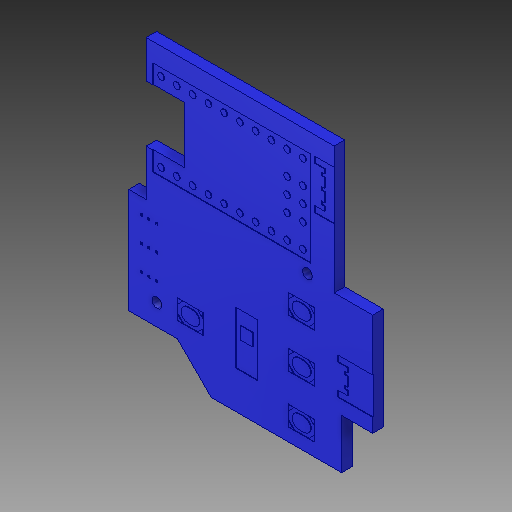
# Autodesk Inventor part: HbBoard
Saved by Autodesk Inventor 2018.1 (Build 221171000, 171)
## iProperties
Part Number: HbBoard
Material: 一般
Document SubType Name: Modeling
Designer: sktom
Density: 1 g/cm^3
Appearance: 青 - 壁塗料 - 光沢
Author: sktom
Autodesk Inventor part; units mm, degrees
ref_plane "YZ Plane" through (0, 0, 0) normal (1, 0, 0) x (0, 1, 0)
ref_plane "XZ Plane" through (0, 0, 0) normal (0, 1, 0) x (-1, 0, 0)
ref_plane "XY Plane" through (0, 0, 0) normal (0, 0, 1) x (1, 0, 0)
sketch "スケッチ1" plane through (0, 0, 0) normal (0, 0, 1) x (1, 0, 0)
  line L0 (-28.6522, -22.804) -> (-22.3388, -22.804) construction
  line L1 (-22.3388, -22.804) -> (-22.3388, -18.1815) construction
  line L2 (-22.3388, -18.1815) -> (-28.6523, -18.1815) construction
  line L3 (-28.6523, -18.1815) -> (-28.6522, -22.804) construction
  circle A0 centre (-24.112, -19.4028) radius 0.5865 construction
  line L4 (-2.2763, -1.725) -> (-2.2763, -4.725) construction
  line L5 (-2.2763, -10.7365) -> (-2.2763, -4.725) construction
  line L6 (-2.2763, -10.7365) -> (2.5447, -10.7365) construction
  line L7 (2.5448, -4.725) -> (2.5447, -10.7365) construction
  line L8 (5.4337, 19.803) -> (5.4337, -0.1035) construction
  line L9 (8.2973, 19.803) -> (5.4337, 19.803) construction
  line L10 (8.2973, 19.803) -> (8.2973, 2.3858) construction
  line L11 (8.2973, 2.3858) -> (7.6738, 2.5529) construction
  ellipse E0 centre (11.2988, 5.779) end of major axis (8.1168, -18.3905) minor radius 3.2094 (7.6738, 2.5529) -> (7.3986, -0.1035) ccw construction
  line L12 (7.3986, -0.1035) -> (5.4337, -0.1035) construction
  line L13 (4.5855, 17.733) -> (-6.16, 17.733) construction
  line L14 (-6.16, 17.733) -> (-17.5935, 17.733) construction
  line L15 (-17.5935, 17.733) -> (-29.1352, 17.733) construction
  spline S0 degree 3 poles (-29.1353, 17.1083) (-29.6143, 16.5272) (-30.1025, 15.9314) (-31.7478, 13.8487) (-32.779, 12.4115) (-34.6914, 9.373) (-35.5322, 7.8351) (-36.9922, 4.7808) (-37.6126, 3.2629) (-38.0872, 1.8206) knots 0.466857 0.466857 0.466857 0.466857 0.772898 0.772898 1.499663 1.499663 2.236131 2.236131 2.977979 2.977979 2.977979 2.977979 construction
  line L16 (-29.5527, 1.5708) -> (-29.5527, -36.2283) construction
  spline S1 degree 3 poles (-29.1127, 5.883) (-29.1127, 6.9607) (-29.1127, 8.0217) (-29.1127, 8.6087) (-29.1127, 9.1968) (-29.1127, 9.2906) (-29.1127, 8.8495) (-29.1127, 8.7808) (-29.1127, 8.7002) (-29.1127, 8.6087) (-29.1127, 8.0217) (-29.1127, 6.9607) (-29.1127, 5.883) knots -1 -1 -1 -1 -0.683333 -0.683333 -0.683333 -0.366056 -0.366056 -0.366056 -0.316667 -0.316667 -0.316667 0 0 0 0 construction
  line L17 (-15.4362, -34.0665) -> (-15.4362, -11.4365) construction
  line L18 (-15.4362, -34.0665) -> (-4.5962, -34.0665) construction
  line L19 (-4.5963, -38.9065) -> (-4.5962, -34.0665) construction
  line L20 (-4.5963, -38.9065) -> (-2.2763, -38.9065) construction
  line L21 (-2.2762, -34.0665) -> (-2.2763, -38.9065) construction
  line L22 (-2.2762, -34.0665) -> (1.7837, -34.0665) construction
  line L23 (1.7838, -11.4365) -> (1.7837, -34.0665) construction
  line L24 (1.7838, -11.4365) -> (-2.2762, -11.4365) construction
  line L25 (-2.2762, -6.5965) -> (-2.2762, -11.4365) construction
  line L26 (-4.5962, -6.5965) -> (-2.2762, -6.5965) construction
  line L27 (-4.5962, -11.4365) -> (-4.5962, -6.5965) construction
  line L28 (-4.5962, -11.4365) -> (-15.4362, -11.4365) construction
  line L29 (-15.4362, -34.0665) -> (-15.4362, -11.4365) construction
  line L30 (-15.4362, -11.4365) -> (-20.9362, -11.4365) construction
  line L31 (-20.9362, -34.0665) -> (-20.9362, -11.4365) construction
  line L32 (-20.9362, -34.0665) -> (-15.4362, -34.0665) construction
  spline S2 degree 3 poles (7.2714, -33.4077) (6.9681, -33.4081) (6.668, -33.4298) (6.3719, -33.4744) (5.9371, -33.5398) (5.5099, -33.6549) (5.0892, -33.8159) (4.6672, -33.9775) (4.2516, -34.1853) (3.8394, -34.4301) (3.381, -34.7024) (2.928, -35.0197) (2.4786, -35.36) (1.9351, -35.7716) (1.3892, -36.2222) (0.8425, -36.6629) (0.2955, -37.1038) (-0.2611, -37.5415) (-0.8412, -37.9413) (-1.2269, -38.2072) (-1.6235, -38.4567) (-2.0345, -38.68) (-2.4446, -38.9027) (-2.869, -39.0994) (-3.3087, -39.2617) (-3.7005, -39.4063) (-4.1048, -39.5234) (-4.518, -39.6095) (-4.7758, -39.6631) (-5.0379, -39.7048) (-5.3012, -39.7342) (-5.3108, -39.7352) (-5.3204, -39.7363) (-5.3299, -39.7373) knots 10.531428 10.531428 10.531428 10.531428 14.175466 14.175466 14.175466 19.526667 19.526667 19.526667 24.893879 24.893879 24.893879 30.861347 30.861347 30.861347 38.077546 38.077546 38.077546 45.296858 45.296858 45.296858 50.098281 50.098281 50.098281 54.888769 54.888769 54.888769 59.156793 59.156793 59.156793 61.818966 61.818966 61.818966 61.915662 61.915662 61.915662 61.915662 construction
  line L33 (-28.8363, -25.7715) -> (-28.8363, -23.7015) construction
  line L34 (-28.8363, -23.7015) -> (-21.3383, -23.7015) construction
  line L35 (-21.3383, -23.7015) -> (-14.7833, -30.2565) construction
  line L36 (-14.7833, -30.2565) -> (5.2957, -30.2565) construction
  line L37 (5.2957, -30.2565) -> (5.2957, -32.3265) construction
  line L38 (5.2957, -32.3265) -> (-15.6802, -32.3265) construction
  line L39 (-15.6802, -32.3265) -> (-22.2353, -25.7715) construction
  line L40 (-28.8363, -25.7715) -> (-22.2353, -25.7715) construction
  circle A1 centre (2.3288, -0.345) radius 0.8
  circle A2 centre (-24.112, -19.4028) radius 0.8
  line L41 (-28.6522, -22.804) -> (-28.6522, -5.867)
  line L42 (-28.6522, -5.867) -> (-25.8627, -5.867)
  line L43 (-25.8627, -5.867) -> (-25.8627, 16.733)
  line L44 (-25.8627, 16.733) -> (5.9172, 16.733)
  line L45 (5.9172, 16.733) -> (5.9172, -3.76)
  line L46 (6.9172, -2.76) -> (10.0274, -2.76) construction
  line L47 (11.6437, -2.76) -> (11.6437, -7.2923) construction
  line L48 (11.6437, -10.3927) -> (11.6437, -2.76) construction
  line L49 (11.2987, -28.1865) -> (11.2987, -18.5265) construction
  line L50 (5.9172, -3.76) -> (10.6437, -3.76)
  line L51 (10.6437, -3.76) -> (10.6437, -28.2565)
  line L52 (10.6437, -28.2565) -> (-15.369, -28.2565)
  line L53 (-15.369, -28.2565) -> (-20.8215, -22.804)
  line L54 (-20.8215, -22.804) -> (-28.6522, -22.804)
  line L55 (-25.8627, 2.2888) -> (-25.8627, 16.733) construction
  line L56 (-8.1718, -5.867) -> (-25.3627, -5.867) construction
  line L57 (6.9172, -2.76) -> (6.9172, 11.3672) construction
  circle A3 centre (0.1342, -3.225) radius 0.55
  line L58 (-2.2763, -4.725) -> (2.5448, -4.725)
  line L59 (2.5448, -4.725) -> (2.5447, -1.725)
  line L60 (2.5448, -4.725) -> (-2.2763, -4.725)
  line L61 (2.5447, -1.725) -> (-2.2763, -1.725)
  point P0 (0, 0)
  point P1 (-17.9831, -31.2915)
  dimension "d0" = 1.6
  dimension "d1" = 1.6
  dimension "d3" = 1
  dimension "d4" = 1
  dimension "d5" = 1
  dimension "d6" = 1
  dimension "d7" = 2
  dimension "d8" = 1
  constraints: 20 end point, 3 horizontal, 3 parallel, 2 centre point, 2 perpendicular, 1 coincident, 1 horizontal alignment, 1 vertical, 1 vertical alignment, 2 other
  measures "d0" diameter of A1
  measures "d1" diameter of A2
  measures "d3" distance between parallel lines of L44 L15
  measures "d4" distance between parallel lines of L57 L45
  measures "d5" distance between parallel lines of L46 L50
  measures "d6" distance between parallel lines of L48 L51
  measures "d7" distance between parallel lines of L36 L52
  measures "d8" distance between parallel lines of L35 L53
extrude "押し出し1" add sketch "スケッチ1" along normal blind 1.7 contours L41 L42 L43 L44 L45 L50 L51 L52 L53 L54 | A3
sketch "スケッチ2" plane through (0, 0, 1.7) normal (0, 0, 1) x (1, 0, 0)
  line L0 (10.6437, -28.2565) -> (10.6437, -3.76) projected
  line L1 (10.6437, -28.2565) -> (5.6437, -28.2565)
  line L2 (10.6437, -28.2565) -> (-15.369, -28.2565) projected
  line L3 (5.6437, -28.2565) -> (5.6437, -20.2565)
  line L4 (5.6437, -20.2565) -> (10.6437, -20.2565)
  line L5 (10.6437, -20.2565) -> (10.6437, -28.2565)
  point P0 (0, 0)
  dimension "d11" = 8
  dimension "d12" = 5
  constraints: 8 end point, 1 horizontal, 1 parallel, 1 point on line, 1 vertical
  measures "d11" distance of L1.end L3.end
  measures "d12" distance of L0.start L1.end
extrude "押し出し2" cut sketch "スケッチ2" against normal blind 1.7
sketch "スケッチ3" plane through (0, 0, 1.7) normal (0, 0, 1) x (1, 0, 0)
  circle A0 centre (0.1342, -3.225) radius 0.55 construction
  circle A1 centre (0.1342, -3.225) radius 0.8
  point P0 (0, 0)
  dimension "d15" = 1.6
  constraints: 1 centre point, 1 coincident
  measures "d15" diameter of A1
extrude "押し出し3" cut sketch "スケッチ3" against normal blind 1.7
delete faces "削除1" heal yes whole lump no faces at (3.1262, -0.4094, 1.1333)
sketch "スケッチ4" plane through (-25.8627, 16.733, 1.7) normal (0, 0, 1) x (1, 0, 0)
  circle A0 centre (5.81, -8.08) radius 0.51 construction
  circle A1 centre (5.81, -10.62) radius 0.51 construction
  circle A2 centre (5.81, -13.16) radius 0.51 construction
  circle A3 centre (5.81, -4.27) radius 0.51 construction
  circle A4 centre (10.89, -4.27) radius 0.51 construction
  circle A5 centre (15.97, -4.27) radius 0.51 construction
  circle A6 centre (21.05, -4.27) radius 0.51 construction
  circle A7 centre (26.13, -4.27) radius 0.51 construction
  circle A8 centre (5.81, -16.97) radius 0.51 construction
  circle A9 centre (10.89, -16.97) radius 0.51 construction
  circle A10 centre (15.97, -16.97) radius 0.51 construction
  circle A11 centre (21.05, -16.97) radius 0.51 construction
  circle A12 centre (26.13, -16.97) radius 0.51 construction
  circle A13 centre (23.59, -16.97) radius 0.51 construction
  circle A14 centre (18.51, -16.97) radius 0.51 construction
  circle A15 centre (13.43, -16.97) radius 0.51 construction
  circle A16 centre (8.35, -16.97) radius 0.51 construction
  circle A17 centre (3.27, -16.97) radius 0.51 construction
  circle A18 centre (23.59, -4.27) radius 0.51 construction
  circle A19 centre (18.51, -4.27) radius 0.51 construction
  circle A20 centre (13.43, -4.27) radius 0.51 construction
  circle A21 centre (8.35, -4.27) radius 0.51 construction
  circle A22 centre (3.27, -4.27) radius 0.51 construction
  circle A23 centre (3.27, -13.16) radius 0.51 construction
  circle A24 centre (3.27, -10.62) radius 0.51 construction
  circle A25 centre (3.27, -8.08) radius 0.51 construction
  line L0 (2, -18.24) -> (2, -3) construction
  line L1 (27.4, -18.24) -> (2, -18.24) construction
  line L2 (27.4, -3) -> (27.4, -18.24) construction
  line L3 (2, -3) -> (27.4, -3) construction
  line L4 (27.4, -6.57) -> (27.4, -14.67) construction
  line L5 (28.5, -14.67) -> (27.4, -14.67) construction
  line L6 (28.5, -6.57) -> (28.5, -14.67) construction
  line L7 (27.4, -6.57) -> (28.5, -6.57) construction
  line L8 (22.9, -14.67) -> (27.4, -14.67) construction
  line L9 (22.9, -6.57) -> (22.9, -14.67) construction
  line L10 (31.78, -17.07) -> (28, -17.07)
  line L11 (28, -17.07) -> (28, -15.07)
  line L12 (28, -15.07) -> (22.5, -15.07)
  line L13 (22.5, -15.07) -> (22.5, -6.17)
  line L14 (22.5, -6.17) -> (28, -6.17)
  line L15 (28, -6.17) -> (28, 0)
  line L16 (31.78, 0) -> (0, 0) projected
  line L17 (31.78, 0) -> (31.78, -17.07)
  point P0 (25.8627, -16.733)
  dimension "d18" = 0.4
  dimension "d19" = 0.4
  dimension "d20" = 0.4
  dimension "d21" = 0.6
  dimension "d22" = 2
  constraints: 14 end point, 5 perpendicular, 3 point on line, 1 horizontal
  measures "d18" distance between parallel lines of L8 L12
  measures "d19" distance between parallel lines of L9 L13
  measures "d20" distance between parallel lines of L7 L14
  measures "d21" distance between parallel lines of L2 L15
  measures "d22" distance of L10.end L11.end
extrude "押し出し4" cut sketch "スケッチ4" against normal blind 1.7
sketch "スケッチ5" plane through (-15.369, -28.2565, 1.7) normal (0, 0, 1) x (1, 0, 0)
  line L0 (26.0128, 24.4965) -> (21.2863, 24.4965) projected
  line L1 (17.5063, 27.9195) -> (17.5063, 29.9195) projected
  line L2 (21.2863, 24.4965) -> (17.5063, 24.4965)
  line L3 (17.5063, 24.4965) -> (17.5063, 27.9195)
  line L4 (17.5063, 27.9195) -> (21.2863, 27.9195)
  line L5 (21.2863, 27.9195) -> (21.2863, 24.4965)
  point P0 (15.369, 28.2565)
  constraints: 8 end point, 2 parallel, 1 horizontal, 1 perpendicular
extrude "押し出し5" cut sketch "スケッチ5" against normal blind 1.7
sketch "スケッチ6" plane through (-15.369, -28.2565, 1.7) normal (0, 0, 1) x (1, 0, 0)
  line L0 (-10.4937, 44.9895) -> (17.5063, 44.9895) projected
  line L1 (17.5063, 44.9895) -> (19.8063, 44.9895)
  line L2 (19.8063, 44.9895) -> (19.8063, 24.4965)
  line L3 (17.5063, 24.4965) -> (26.0128, 24.4965) projected
  line L4 (17.5063, 38.8195) -> (17.5063, 44.9895) projected
  line L5 (17.5063, 29.9195) -> (17.5063, 24.4965) projected
  line L6 (19.8063, 24.4965) -> (17.5063, 24.4965)
  line L7 (17.5063, 24.4965) -> (17.5063, 29.9195)
  line L8 (12.0063, 29.9195) -> (12.0063, 38.8195) projected
  line L9 (17.5063, 29.9195) -> (12.0063, 29.9195)
  line L10 (12.0063, 29.9195) -> (12.0063, 38.8195)
  line L11 (17.5063, 38.8195) -> (12.0063, 38.8195) projected
  line L12 (12.0063, 38.8195) -> (17.5063, 38.8195)
  line L13 (17.5063, 38.8195) -> (17.5063, 44.9895)
  point P0 (15.369, 28.2565)
  dimension "d27" = 2.3
  constraints: 16 end point, 6 perpendicular, 1 collinear, 1 horizontal, 1 point on line
  measures "d27" distance between parallel lines of L4 L2
extrude "押し出し6" add sketch "スケッチ6" against normal up to surface (1.7 mm away)
sketch "スケッチ7" plane through (-15.369, -28.2565, 1.7) normal (0, 0, 1) x (1, 0, 0)
  line L0 (-9.3937, 30.3195) -> (-9.3937, 38.4195) projected
  line L1 (-10.4937, 38.4195) -> (-9.3937, 38.4195) projected
  line L2 (-10.4937, 30.3195) -> (-10.4937, 38.4195) projected
  line L3 (-9.3937, 30.3195) -> (-10.4937, 30.3195) projected
  line L4 (-4.8937, 30.3195) -> (-4.8937, 38.4195) projected
  line L5 (-10.9937, 38.9195) -> (-4.3937, 38.9195)
  line L6 (-4.3937, 38.9195) -> (-4.3937, 29.8195)
  line L7 (-4.3937, 29.8195) -> (-10.9937, 29.8195)
  line L8 (-10.9937, 29.8195) -> (-10.9937, 38.9195)
  point P0 (15.369, 28.2565)
  dimension "d30" = 0.5
  dimension "d31" = 0.5
  dimension "d32" = 0.5
  dimension "d33" = 0.5
  constraints: 8 end point, 2 parallel, 1 horizontal, 1 perpendicular
  measures "d30" distance between parallel lines of L6 L4
  measures "d31" distance between parallel lines of L3 L7
  measures "d32" distance between parallel lines of L1 L5
  measures "d33" distance between parallel lines of L2 L8
extrude "押し出し7" cut sketch "スケッチ7" against normal blind 10 contours L3 L2 L1 L0 | L5 L6 L7 L8
sketch "スケッチ8" plane through (-15.369, -28.2565, 1.7) normal (0, 0, 1) x (1, 0, 0)
  line L0 (22.0128, 11.93) -> (21.5128, 11.93) projected
  line L1 (22.0128, 12.43) -> (22.0128, 11.93) projected
  line L2 (21.5128, 12.43) -> (22.0128, 12.43) projected
  line L3 (21.5128, 11.93) -> (21.5128, 12.43) projected
  line L4 (22.0128, 13.93) -> (21.5128, 13.93) projected
  line L5 (22.0128, 14.43) -> (22.0128, 13.93) projected
  line L6 (21.5128, 14.43) -> (22.0128, 14.43) projected
  line L7 (21.5128, 13.93) -> (21.5128, 14.43) projected
  line L8 (16.5666, 9.924) -> (15.7166, 9.924) projected
  line L9 (15.7166, 9.924) -> (16.5666, 10.774) projected
  line L10 (16.5666, 10.774) -> (16.5666, 9.924) projected
  line L11 (13.3166, 9.924) -> (12.4666, 9.924) projected
  line L12 (12.4666, 9.924) -> (12.4666, 10.774) projected
  line L13 (12.4666, 10.774) -> (13.3166, 9.924) projected
  line L14 (15.7166, 13.024) -> (16.5666, 13.024) projected
  line L15 (16.5666, 13.024) -> (16.5666, 12.174) projected
  line L16 (16.5666, 12.174) -> (15.7166, 13.024) projected
  line L17 (12.4666, 13.024) -> (13.3166, 13.024) projected
  line L18 (13.3166, 13.024) -> (12.4666, 12.174) projected
  line L19 (12.4666, 12.174) -> (12.4666, 13.024) projected
  arc A0 (14.1166, 12.574) -> (14.1166, 10.374) centre (14.1166, 11.474) ccw projected
  line L20 (14.1166, 12.574) -> (14.9166, 12.574) projected
  arc A1 (14.9166, 10.374) -> (14.9166, 12.574) centre (14.9166, 11.474) ccw projected
  line L21 (14.9166, 10.374) -> (14.1166, 10.374) projected
  line L22 (12.4166, 9.874) -> (16.6166, 9.874) projected
  line L23 (16.6166, 9.874) -> (16.6166, 13.074) projected
  line L24 (16.6166, 13.074) -> (12.4166, 13.074) projected
  line L25 (12.4166, 13.074) -> (12.4166, 9.874) projected
  line L26 (16.5666, 2.124) -> (15.7166, 2.124) projected
  line L27 (15.7166, 2.124) -> (16.5666, 2.974) projected
  line L28 (16.5666, 2.974) -> (16.5666, 2.124) projected
  line L29 (13.3166, 2.124) -> (12.4666, 2.124) projected
  line L30 (12.4666, 2.124) -> (12.4666, 2.974) projected
  line L31 (12.4666, 2.974) -> (13.3166, 2.124) projected
  line L32 (15.7166, 5.224) -> (16.5666, 5.224) projected
  line L33 (16.5666, 5.224) -> (16.5666, 4.374) projected
  line L34 (16.5666, 4.374) -> (15.7166, 5.224) projected
  line L35 (12.4666, 5.224) -> (13.3166, 5.224) projected
  line L36 (13.3166, 5.224) -> (12.4666, 4.374) projected
  line L37 (12.4666, 4.374) -> (12.4666, 5.224) projected
  arc A2 (14.1166, 4.774) -> (14.1166, 2.574) centre (14.1166, 3.674) ccw projected
  line L38 (14.1166, 4.774) -> (14.9166, 4.774) projected
  arc A3 (14.9166, 2.574) -> (14.9166, 4.774) centre (14.9166, 3.674) ccw projected
  line L39 (14.9166, 2.574) -> (14.1166, 2.574) projected
  line L40 (12.4166, 2.074) -> (16.6166, 2.074) projected
  line L41 (16.6166, 2.074) -> (16.6166, 5.274) projected
  line L42 (16.6166, 5.274) -> (12.4166, 5.274) projected
  line L43 (12.4166, 5.274) -> (12.4166, 2.074) projected
  line L44 (16.5666, 17.724) -> (15.7166, 17.724) projected
  line L45 (15.7166, 17.724) -> (16.5666, 18.574) projected
  line L46 (16.5666, 18.574) -> (16.5666, 17.724) projected
  line L47 (13.3166, 17.724) -> (12.4666, 17.724) projected
  line L48 (12.4666, 17.724) -> (12.4666, 18.574) projected
  line L49 (12.4666, 18.574) -> (13.3166, 17.724) projected
  line L50 (15.7166, 20.824) -> (16.5666, 20.824) projected
  line L51 (16.5666, 20.824) -> (16.5666, 19.974) projected
  line L52 (16.5666, 19.974) -> (15.7166, 20.824) projected
  line L53 (12.4666, 20.824) -> (13.3166, 20.824) projected
  line L54 (13.3166, 20.824) -> (12.4666, 19.974) projected
  line L55 (12.4666, 19.974) -> (12.4666, 20.824) projected
  arc A4 (14.1166, 20.374) -> (14.1166, 18.174) centre (14.1166, 19.274) ccw projected
  line L56 (14.1166, 20.374) -> (14.9166, 20.374) projected
  arc A5 (14.9166, 18.174) -> (14.9166, 20.374) centre (14.9166, 19.274) ccw projected
  line L57 (14.9166, 18.174) -> (14.1166, 18.174) projected
  line L58 (12.4166, 17.674) -> (16.6166, 17.674) projected
  line L59 (16.6166, 17.674) -> (16.6166, 20.874) projected
  line L60 (16.6166, 20.874) -> (12.4166, 20.874) projected
  line L61 (12.4166, 20.874) -> (12.4166, 17.674) projected
  line L62 (-1.2944, 11.1885) -> (-5.4944, 11.1885) projected
  line L63 (-1.3444, 8.0385) -> (-2.1944, 8.0385) projected
  line L64 (-2.1944, 8.0385) -> (-1.3444, 8.8885) projected
  line L65 (-1.3444, 8.8885) -> (-1.3444, 8.0385) projected
  line L66 (-4.5944, 8.0385) -> (-5.4444, 8.0385) projected
  line L67 (-5.4444, 8.0385) -> (-5.4444, 8.8885) projected
  line L68 (-5.4444, 8.8885) -> (-4.5944, 8.0385) projected
  line L69 (-2.1944, 11.1385) -> (-1.3444, 11.1385) projected
  line L70 (-1.3444, 11.1385) -> (-1.3444, 10.2885) projected
  line L71 (-1.3444, 10.2885) -> (-2.1944, 11.1385) projected
  line L72 (-5.4444, 11.1385) -> (-4.5944, 11.1385) projected
  line L73 (-4.5944, 11.1385) -> (-5.4444, 10.2885) projected
  line L74 (-5.4444, 10.2885) -> (-5.4444, 11.1385) projected
  arc A6 (-3.7944, 10.6885) -> (-3.7944, 8.4885) centre (-3.7944, 9.5885) ccw projected
  line L75 (-3.7944, 10.6885) -> (-2.9944, 10.6885) projected
  arc A7 (-2.9944, 8.4885) -> (-2.9944, 10.6885) centre (-2.9944, 9.5885) ccw projected
  line L76 (-2.9944, 8.4885) -> (-3.7944, 8.4885) projected
  line L77 (-5.4944, 7.9885) -> (-1.2944, 7.9885) projected
  line L78 (-1.2944, 7.9885) -> (-1.2944, 11.1885) projected
  line L79 (-1.2944, 11.1885) -> (-5.4944, 11.1885) projected
  line L80 (-5.4944, 11.1885) -> (-5.4944, 7.9885) projected
  line L81 (4.6778, 10.3689) -> (4.6778, 12.3689) projected
  line L82 (4.6778, 12.3689) -> (6.6778, 12.3689) projected
  line L83 (6.6778, 12.3689) -> (6.6778, 10.3689) projected
  line L84 (6.6778, 10.3689) -> (4.6778, 10.3689) projected
  line L85 (3.9278, 6.0689) -> (7.4278, 6.0689) projected
  line L86 (7.4278, 6.0689) -> (7.4278, 14.5689) projected
  line L87 (7.4278, 14.5689) -> (3.9278, 14.5689) projected
  line L88 (3.9278, 14.5689) -> (3.9278, 6.0689) projected
  circle A8 centre (12.1963, 31.8295) radius 0.51 projected
  circle A9 centre (12.1963, 34.3695) radius 0.51 projected
  circle A10 centre (12.1963, 36.9095) radius 0.51 projected
  circle A11 centre (12.1963, 28.0195) radius 0.51 projected
  circle A12 centre (7.1163, 28.0195) radius 0.51 projected
  circle A13 centre (2.0363, 28.0195) radius 0.51 projected
  circle A14 centre (-3.0437, 28.0195) radius 0.51 projected
  circle A15 centre (-8.1237, 28.0195) radius 0.51 projected
  circle A16 centre (12.1963, 40.7195) radius 0.51 projected
  circle A17 centre (7.1163, 40.7195) radius 0.51 projected
  circle A18 centre (2.0363, 40.7195) radius 0.51 projected
  circle A19 centre (-3.0437, 40.7195) radius 0.51 projected
  circle A20 centre (-8.1237, 40.7195) radius 0.51 projected
  circle A21 centre (-5.5837, 40.7195) radius 0.51 projected
  circle A22 centre (-0.5037, 40.7195) radius 0.51 projected
  circle A23 centre (4.5763, 40.7195) radius 0.51 projected
  circle A24 centre (9.6563, 40.7195) radius 0.51 projected
  circle A25 centre (14.7363, 40.7195) radius 0.51 projected
  circle A26 centre (-5.5837, 28.0195) radius 0.51 projected
  circle A27 centre (-0.5037, 28.0195) radius 0.51 projected
  circle A28 centre (4.5763, 28.0195) radius 0.51 projected
  circle A29 centre (9.6563, 28.0195) radius 0.51 projected
  circle A30 centre (14.7363, 28.0195) radius 0.51 projected
  circle A31 centre (14.7363, 36.9095) radius 0.51 projected
  circle A32 centre (14.7363, 34.3695) radius 0.51 projected
  circle A33 centre (14.7363, 31.8295) radius 0.51 projected
  line L89 (16.0063, 41.9895) -> (16.0063, 26.7495) projected
  line L90 (-9.3937, 41.9895) -> (16.0063, 41.9895) projected
  line L91 (-9.3937, 26.7495) -> (-9.3937, 41.9895) projected
  line L92 (16.0063, 26.7495) -> (-9.3937, 26.7495) projected
  line L93 (18.2863, 35.821) -> (17.7863, 35.821) projected
  line L94 (18.2863, 36.321) -> (18.2863, 35.821) projected
  line L95 (17.7863, 36.321) -> (18.2863, 36.321) projected
  line L96 (17.7863, 35.821) -> (17.7863, 36.321) projected
  line L97 (18.2863, 37.821) -> (17.7863, 37.821) projected
  line L98 (18.2863, 38.321) -> (18.2863, 37.821) projected
  line L99 (17.7863, 38.321) -> (18.2863, 38.321) projected
  line L100 (17.7863, 37.821) -> (17.7863, 38.321) projected
  line L101 (18.7328, 29.2915) -> (18.7328, 45.9895) projected
  line L102 (18.2863, 39.821) -> (17.7863, 39.821) projected
  line L103 (18.2863, 40.321) -> (18.2863, 39.821) projected
  line L104 (17.7863, 40.321) -> (18.2863, 40.321) projected
  line L105 (17.7863, 39.821) -> (17.7863, 40.321) projected
  line L106 (18.2863, 41.021) -> (18.2863, 40.321) projected
  line L107 (18.2863, 40.321) -> (18.2863, 39.821) projected
  line L108 (18.2863, 39.821) -> (18.2863, 38.321) projected
  line L109 (18.2863, 38.321) -> (18.2863, 37.821) projected
  line L110 (18.2863, 37.821) -> (18.2863, 36.321) projected
  line L111 (18.2863, 36.321) -> (18.2863, 35.821) projected
  line L112 (18.2863, 35.821) -> (18.2863, 35.121) projected
  line L113 (18.2863, 35.121) -> (16.6863, 35.121) projected
  line L114 (16.6863, 34.121) -> (16.6863, 35.121) projected
  line L115 (24.2863, 34.121) -> (16.6863, 34.121) projected
  line L116 (24.2863, 34.121) -> (24.2863, 42.021) projected
  line L117 (24.2863, 42.021) -> (16.6863, 42.021) projected
  line L118 (16.6863, 41.021) -> (16.6863, 42.021) projected
  line L119 (16.6863, 41.021) -> (18.2863, 41.021) projected
  line L120 (-11.4432, 20.0251) -> (-11.3332, 19.9151) projected
  line L121 (-11.4432, 20.0251) -> (-11.4432, 19.6751) projected
  line L122 (-11.4432, 19.6751) -> (-11.3332, 19.7851) projected
  line L123 (-11.3332, 19.9151) -> (-11.3332, 19.7851) projected
  line L124 (-11.4432, 20.0251) -> (-11.3332, 19.9151) projected
  line L125 (-11.2332, 19.9151) -> (-11.3332, 19.9151) projected
  line L126 (-11.1232, 20.0251) -> (-11.2332, 19.9151) projected
  line L127 (-11.1232, 20.0251) -> (-11.4432, 20.0251) projected
  line L128 (-11.1232, 20.0251) -> (-11.2332, 19.9151) projected
  line L129 (-11.2332, 19.7851) -> (-11.2332, 19.9151) projected
  line L130 (-11.1232, 19.6751) -> (-11.2332, 19.7851) projected
  line L131 (-11.1232, 19.6751) -> (-11.1232, 20.0251) projected
  line L132 (-11.4432, 19.6751) -> (-11.3332, 19.7851) projected
  line L133 (-11.4432, 19.6751) -> (-11.1232, 19.6751) projected
  line L134 (-11.1232, 19.6751) -> (-11.2332, 19.7851) projected
  line L135 (-11.3332, 19.7851) -> (-11.2332, 19.7851) projected
  line L136 (-10.1932, 19.6751) -> (-10.0832, 19.7851) projected
  line L137 (-10.1932, 19.6751) -> (-9.8732, 19.6751) projected
  line L138 (-9.8732, 19.6751) -> (-9.9832, 19.7851) projected
  line L139 (-10.0832, 19.7851) -> (-9.9832, 19.7851) projected
  line L140 (-9.8732, 20.0251) -> (-9.9832, 19.9151) projected
  line L141 (-9.9832, 19.7851) -> (-9.9832, 19.9151) projected
  line L142 (-9.8732, 19.6751) -> (-9.9832, 19.7851) projected
  line L143 (-9.8732, 19.6751) -> (-9.8732, 20.0251) projected
  line L144 (-10.1932, 20.0251) -> (-10.0832, 19.9151) projected
  line L145 (-10.1932, 20.0251) -> (-10.1932, 19.6751) projected
  line L146 (-10.1932, 19.6751) -> (-10.0832, 19.7851) projected
  line L147 (-10.0832, 19.9151) -> (-10.0832, 19.7851) projected
  line L148 (-10.1932, 20.0251) -> (-10.0832, 19.9151) projected
  line L149 (-9.9832, 19.9151) -> (-10.0832, 19.9151) projected
  line L150 (-9.8732, 20.0251) -> (-9.9832, 19.9151) projected
  line L151 (-9.8732, 20.0251) -> (-10.1932, 20.0251) projected
  line L152 (-8.9432, 19.6751) -> (-8.6232, 19.6751) projected
  line L153 (-8.6232, 19.6751) -> (-8.7332, 19.7851) projected
  line L154 (-8.8332, 19.7851) -> (-8.7332, 19.7851) projected
  line L155 (-8.9432, 19.6751) -> (-8.8332, 19.7851) projected
  line L156 (-8.9432, 20.0251) -> (-8.9432, 19.6751) projected
  line L157 (-8.9432, 19.6751) -> (-8.8332, 19.7851) projected
  line L158 (-8.8332, 19.9151) -> (-8.8332, 19.7851) projected
  line L159 (-8.9432, 20.0251) -> (-8.8332, 19.9151) projected
  line L160 (-8.7332, 19.7851) -> (-8.7332, 19.9151) projected
  line L161 (-8.6232, 19.6751) -> (-8.7332, 19.7851) projected
  line L162 (-8.6232, 19.6751) -> (-8.6232, 20.0251) projected
  line L163 (-8.6232, 20.0251) -> (-8.7332, 19.9151) projected
  line L164 (-8.7332, 19.9151) -> (-8.8332, 19.9151) projected
  line L165 (-8.6232, 20.0251) -> (-8.7332, 19.9151) projected
  line L166 (-8.6232, 20.0251) -> (-8.9432, 20.0251) projected
  line L167 (-8.9432, 20.0251) -> (-8.8332, 19.9151) projected
  line L168 (-8.9432, 15.6751) -> (-8.6232, 15.6751) projected
  line L169 (-8.6232, 15.6751) -> (-8.7332, 15.7851) projected
  line L170 (-8.8332, 15.7851) -> (-8.7332, 15.7851) projected
  line L171 (-8.9432, 15.6751) -> (-8.8332, 15.7851) projected
  line L172 (-8.7332, 15.7851) -> (-8.7332, 15.9151) projected
  line L173 (-8.6232, 15.6751) -> (-8.7332, 15.7851) projected
  line L174 (-8.6232, 15.6751) -> (-8.6232, 16.0251) projected
  line L175 (-8.6232, 16.0251) -> (-8.7332, 15.9151) projected
  line L176 (-8.7332, 15.9151) -> (-8.8332, 15.9151) projected
  line L177 (-8.6232, 16.0251) -> (-8.7332, 15.9151) projected
  line L178 (-8.6232, 16.0251) -> (-8.9432, 16.0251) projected
  line L179 (-8.9432, 16.0251) -> (-8.8332, 15.9151) projected
  line L180 (-8.9432, 16.0251) -> (-8.9432, 15.6751) projected
  line L181 (-8.9432, 15.6751) -> (-8.8332, 15.7851) projected
  line L182 (-8.8332, 15.9151) -> (-8.8332, 15.7851) projected
  line L183 (-8.9432, 16.0251) -> (-8.8332, 15.9151) projected
  line L184 (-9.8732, 16.0251) -> (-9.9832, 15.9151) projected
  line L185 (-9.9832, 15.7851) -> (-9.9832, 15.9151) projected
  line L186 (-9.8732, 15.6751) -> (-9.9832, 15.7851) projected
  line L187 (-9.8732, 15.6751) -> (-9.8732, 16.0251) projected
  line L188 (-10.1932, 15.6751) -> (-10.0832, 15.7851) projected
  line L189 (-10.1932, 15.6751) -> (-9.8732, 15.6751) projected
  line L190 (-9.8732, 15.6751) -> (-9.9832, 15.7851) projected
  line L191 (-10.0832, 15.7851) -> (-9.9832, 15.7851) projected
  line L192 (-9.9832, 16.0251) -> (-9.9832, 15.6251) projected
  line L193 (-10.1932, 16.0251) -> (-10.0832, 15.9151) projected
  line L194 (-9.9832, 15.9151) -> (-10.0832, 15.9151) projected
  line L195 (-9.8732, 16.0251) -> (-9.9832, 15.9151) projected
  line L196 (-9.8732, 16.0251) -> (-10.1932, 16.0251) projected
  line L197 (-10.1932, 16.0251) -> (-10.0832, 15.9151) projected
  line L198 (-10.1932, 16.0251) -> (-10.1932, 15.6751) projected
  line L199 (-10.1932, 15.6751) -> (-10.0832, 15.7851) projected
  line L200 (-10.0832, 15.9151) -> (-10.0832, 15.7851) projected
  line L201 (-11.1232, 16.0251) -> (-11.2332, 15.9151) projected
  line L202 (-11.2332, 15.7851) -> (-11.2332, 15.9151) projected
  line L203 (-11.1232, 15.6751) -> (-11.2332, 15.7851) projected
  line L204 (-11.1232, 15.6751) -> (-11.1232, 16.0251) projected
  line L205 (-11.4432, 15.6751) -> (-11.3332, 15.7851) projected
  line L206 (-11.4432, 15.6751) -> (-11.1232, 15.6751) projected
  line L207 (-11.1232, 15.6751) -> (-11.2332, 15.7851) projected
  line L208 (-11.3332, 15.7851) -> (-11.2332, 15.7851) projected
  line L209 (-11.4432, 16.0251) -> (-11.3332, 15.9151) projected
  line L210 (-11.4432, 16.0251) -> (-11.4432, 15.6751) projected
  line L211 (-11.4432, 15.6751) -> (-11.3332, 15.7851) projected
  line L212 (-11.3332, 15.9151) -> (-11.3332, 15.7851) projected
  line L213 (-11.4432, 16.0251) -> (-11.3332, 15.9151) projected
  line L214 (-11.2332, 15.9151) -> (-11.3332, 15.9151) projected
  line L215 (-11.1232, 16.0251) -> (-11.2332, 15.9151) projected
  line L216 (-11.1232, 16.0251) -> (-11.4432, 16.0251) projected
  line L217 (-11.4432, 11.6751) -> (-11.3332, 11.7851) projected
  line L218 (-11.4432, 11.6751) -> (-11.1232, 11.6751) projected
  line L219 (-11.1232, 11.6751) -> (-11.2332, 11.7851) projected
  line L220 (-11.3332, 11.7851) -> (-11.2332, 11.7851) projected
  line L221 (-11.4432, 12.0251) -> (-11.3332, 11.9151) projected
  line L222 (-11.4432, 12.0251) -> (-11.4432, 11.6751) projected
  line L223 (-11.4432, 11.6751) -> (-11.3332, 11.7851) projected
  line L224 (-11.3332, 11.9151) -> (-11.3332, 11.7851) projected
  line L225 (-11.4432, 12.0251) -> (-11.3332, 11.9151) projected
  line L226 (-11.2332, 11.9151) -> (-11.3332, 11.9151) projected
  line L227 (-11.1232, 12.0251) -> (-11.2332, 11.9151) projected
  line L228 (-11.1232, 12.0251) -> (-11.4432, 12.0251) projected
  line L229 (-11.1232, 12.0251) -> (-11.2332, 11.9151) projected
  line L230 (-11.2332, 11.7851) -> (-11.2332, 11.9151) projected
  line L231 (-11.1232, 11.6751) -> (-11.2332, 11.7851) projected
  line L232 (-11.1232, 11.6751) -> (-11.1232, 12.0251) projected
  line L233 (-10.1932, 12.0251) -> (-10.0832, 11.9151) projected
  line L234 (-10.1932, 12.0251) -> (-10.1932, 11.6751) projected
  line L235 (-10.1932, 11.6751) -> (-10.0832, 11.7851) projected
  line L236 (-10.0832, 11.9151) -> (-10.0832, 11.7851) projected
  line L237 (-10.1932, 11.6751) -> (-10.0832, 11.7851) projected
  line L238 (-10.1932, 11.6751) -> (-9.8732, 11.6751) projected
  line L239 (-9.8732, 11.6751) -> (-9.9832, 11.7851) projected
  line L240 (-10.0832, 11.7851) -> (-9.9832, 11.7851) projected
  line L241 (-10.1932, 12.0251) -> (-10.0832, 11.9151) projected
  line L242 (-9.9832, 11.9151) -> (-10.0832, 11.9151) projected
  line L243 (-9.8732, 12.0251) -> (-9.9832, 11.9151) projected
  line L244 (-9.8732, 12.0251) -> (-10.1932, 12.0251) projected
  line L245 (-9.8732, 12.0251) -> (-9.9832, 11.9151) projected
  line L246 (-9.9832, 11.7851) -> (-9.9832, 11.9151) projected
  line L247 (-9.8732, 11.6751) -> (-9.9832, 11.7851) projected
  line L248 (-9.8732, 11.6751) -> (-9.8732, 12.0251) projected
  line L249 (-8.9432, 12.0251) -> (-8.9432, 11.6751) projected
  line L250 (-8.9432, 11.6751) -> (-8.8332, 11.7851) projected
  line L251 (-8.8332, 11.9151) -> (-8.8332, 11.7851) projected
  line L252 (-8.9432, 12.0251) -> (-8.8332, 11.9151) projected
  line L253 (-8.9432, 11.6751) -> (-8.6232, 11.6751) projected
  line L254 (-8.6232, 11.6751) -> (-8.7332, 11.7851) projected
  line L255 (-8.8332, 11.7851) -> (-8.7332, 11.7851) projected
  line L256 (-8.9432, 11.6751) -> (-8.8332, 11.7851) projected
  line L257 (-8.7332, 11.7851) -> (-8.7332, 11.9151) projected
  line L258 (-8.6232, 11.6751) -> (-8.7332, 11.7851) projected
  line L259 (-8.6232, 11.6751) -> (-8.6232, 12.0251) projected
  line L260 (-8.6232, 12.0251) -> (-8.7332, 11.9151) projected
  line L261 (-8.6232, 12.0251) -> (-8.9432, 12.0251) projected
  line L262 (-8.7332, 11.9151) -> (-8.8332, 11.9151) projected
  line L263 (-8.6232, 12.0251) -> (-8.7332, 11.9151) projected
  line L264 (-8.6232, 12.0251) -> (-8.9432, 12.0251) projected
  line L265 (-8.9432, 12.0251) -> (-8.8332, 11.9151) projected
  line L266 (22.0128, 15.13) -> (22.0128, 14.43) projected
  line L267 (22.0128, 14.43) -> (22.0128, 13.93) projected
  line L268 (22.0128, 13.93) -> (22.0128, 12.43) projected
  line L269 (22.0128, 12.43) -> (22.0128, 11.93) projected
  line L270 (22.0128, 11.93) -> (22.0128, 11.23) projected
  line L271 (22.0128, 11.23) -> (20.4128, 11.23) projected
  line L272 (20.4128, 10.23) -> (20.4128, 11.23) projected
  line L273 (28.0128, 10.23) -> (20.4128, 10.23) projected
  line L274 (28.0128, 10.23) -> (28.0128, 16.13) projected
  line L275 (28.0128, 16.13) -> (20.4128, 16.13) projected
  line L276 (20.4128, 15.13) -> (20.4128, 16.13) projected
  line L277 (20.4128, 15.13) -> (22.0128, 15.13) projected
  line L278 (-12.7832, 10.7001) -> (-12.7832, 13.5001) projected
  point P0 (15.369, 28.2565)
extrude "押し出し8" cut sketch "スケッチ8" against normal blind 0.1 contours L0 L3 L2 L1 | L1 L268 L5 L266 L277 L276 L275 L274 L273 L272 L271 L270 | L4 L7 L6 L5 | L25 L24 L23 L22 | L43 L42 L41 L40 | L61 L60 L59 L58 | L78 L77 L80 L62 | L88 L87 L86 L85 | L89 L92 L91 L90 | L93 L96 L95 L94 | L94 L110 L98 L108 L103 L106 L119 L118 L117 L101 L115 L114 L113 L112 | L97 L100 L99 L98 | L102 L105 L104 L103 | L101 L117 L116 L115 | L127 L126 L125 L120 | L120 L123 L122 L121 | L122 L135 L130 L133 | L131 L130 L129 L126 | L145 L144 L147 L136 | L136 L139 L138 L137 | L138 L141 L140 L143 | L151 L140 L149 L144 | L156 L159 L158 L155 | L153 L160 L163 L162 | L166 L163 L164 L159 | L171 L170 L169 L168 | L180 L179 L182 L171 | L169 L172 L175 L174 | L178 L175 L176 L179 | L187 L186 L185 L184 | L184 L192 L196 | L194 L193 L196 L192 | L189 L192 L186 | L192 L189 L188 L191 | L200 L188 L198 L193 | L204 L203 L202 L201 | L201 L214 L209 L216 | L206 L205 L208 L203 | L209 L212 L205 L210 | L222 L221 L224 L217 | L217 L220 L219 L218 | L219 L230 L227 L232 | L228 L227 L226 L221 | L244 L243 L242 L233 | L233 L236 L235 L234 | L235 L240 L239 L238 | L248 L239 L246 L243 | L252 L251 L250 L249 | L261 L260 L262 L252 | L250 L255 L254 L253 | L259 L254 L257 L260
